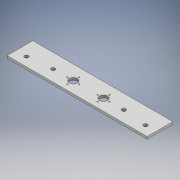
# Autodesk Inventor part: 1021sidemotorN
Saved by Autodesk Inventor 2017 (Build 210142000, 142)
## iProperties
Created: 2016-10-15
Part Number: 1021sidemotorN
Material: Generic
Document SubType Name: Modeling
Designer: Kevin G
Density: 1 g/cm^3
Appearance: Default
Author: Kevin G
Autodesk Inventor part; units mm, degrees
ref_plane "YZ Plane" through (0, 0, 0) normal (1, 0, 0) x (0, 1, 0)
ref_plane "XZ Plane" through (0, 0, 0) normal (0, 1, 0) x (-1, 0, 0)
ref_plane "XY Plane" through (0, 0, 0) normal (0, 0, 1) x (1, 0, 0)
sketch "Sketch1" plane through (0, 0, 0) normal (0, 0, 1) x (1, 0, 0)
  line L0 (-270.2344, -114.33) -> (-270.2344, -13.08)
  line L1 (-238, -114.33) -> (-238, -79.405)
  circle A0 centre (-228.9594, -79.405) radius 7.5
  line L2 (-141, -114.33) -> (-141, -69.88)
  circle A1 centre (-133.7094, -69.88) radius 7.5
  circle A2 centre (-54.3344, -69.88) radius 15.875
  circle A3 centre (-54.3344, -46.8612) radius 2.3813
  circle A4 centre (-31.3157, -69.88) radius 2.3813
  circle A5 centre (-77.3532, -69.88) radius 2.3813
  circle A6 centre (-54.3344, -92.8987) radius 2.3813
  line L3 (-270.2344, -13.08) -> (5.175, -13.08)
  line L4 (-270.2344, -114.33) -> (5.1968, -114.33)
  line L5 (280.6281, -114.33) -> (280.6281, -13.08)
  circle A7 centre (239.3531, -79.405) radius 7.5
  circle A8 centre (144.1031, -69.88) radius 7.5
  circle A9 centre (64.7281, -69.88) radius 15.875
  circle A10 centre (64.7281, -46.8612) radius 2.3813
  circle A11 centre (41.7093, -69.88) radius 2.3813
  circle A12 centre (87.7468, -69.88) radius 2.3813
  circle A13 centre (64.7281, -92.8987) radius 2.3813
  line L6 (280.6281, -13.08) -> (5.175, -13.08)
  line L7 (280.6281, -114.33) -> (5.1968, -114.33)
  point P0 (2, -13.08)
  point P1 (2, -114.33)
  point P2 (-270.2344, -56.825)
  point P3 (-270.2344, -60)
  point P4 (280.6281, -56.825)
  point P5 (280.6281, -60)
  dimension "d3" = 34.925
  dimension "d4" = 15
  dimension "d6" = 44.45
  dimension "d7" = 15
  dimension "d9" = 31.75
  dimension "d11" = 4.7625
  dimension "d13" = 4.7625
  dimension "d15" = 23.0188
  dimension "d16" = 4.7625
  dimension "d18" = 4.7625
  dimension "d23" = 79.375
  dimension "d44" = 15
  dimension "d45" = 15
  constraints: 16 end point, 14 centre point, 6 point on line, 2 vertical, 1 horizontal
  measures "d3" distance of L1.start L1.end
  measures "d4" diameter of A0
  measures "d6" distance of L2.end L2.start
  measures "d7" diameter of A1
  measures "d9" diameter of A2
  measures "d11" diameter of A3
  measures "d13" diameter of A4
  measures "d15" distance of A2.centre A5.centre
  measures "d16" diameter of A5
  measures "d18" diameter of A6
  measures "d23" distance of A8.centre A9.centre
  measures "d44" diameter of A8
  measures "d45" diameter of A7
extrude "Extrusion2" add sketch "Sketch1" along normal blind 9.525
body "Solid2"
